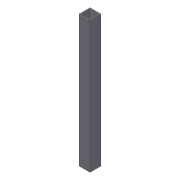
# Autodesk Inventor part: Frame_FrontVerticalShooterSupport
Saved by Autodesk Inventor 2012 (Build 160160000, 160)
## iProperties
Created: 2012-01-21
Part Number: Frame_FrontVerticalShooterSupport
Material: Aluminum-6061
Document SubType Name: Modeling
Designer: JesseK
Mass: 124.9 g
Surface Area: 583.668 cm^2
Volume: 46.0886 cm^3
Density: 2.71 g/cm^3
Author: JesseK
Autodesk Inventor part; units mm, degrees
ref_plane "YZ Plane" through (0, 0, 0) normal (1, 0, 0) x (0, 1, 0)
ref_plane "XZ Plane" through (0, 0, 0) normal (0, 1, 0) x (-1, 0, 0)
ref_plane "XY Plane" through (0, 0, 0) normal (0, 0, 1) x (1, 0, 0)
sketch "Sketch1" plane through (0, 0, 0) normal (0, 0, 1) x (1, 0, 0)
  line L0 (0, 0) -> (25.4, 0)
  line L1 (25.4, 0) -> (25.4, 304.8)
  line L2 (25.4, 304.8) -> (0, 304.8)
  line L3 (0, 304.8) -> (0, 0)
  dimension "d0" = 25.4
  dimension "d1" = 304.8
  constraints: 8 end point, 2 parallel, 1 horizontal, 1 perpendicular
  measures "d0" distance of L0.start L0.end
  measures "d1" distance of L2.end L0.start
extrude "Extrusion1" add sketch "Sketch1" along normal blind 25.4
shell "Shell1" thickness 1.5875 removed faces 2 at (16.9333, 304.8, 8.4667) at (8.4667, 0, 8.4667)
body "Solid1"
